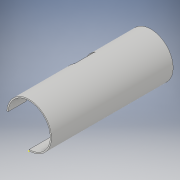
# Autodesk Inventor part: upperClaw
Saved by Autodesk Inventor 2017 (Build 210142000, 142)
## iProperties
Created: 2017-04-06
Part Number: upperClaw
Material: Generic
Document SubType Name: Modeling
Designer: s4461999
Density: 1 g/cm^3
Appearance: Default
Author: s4461999
Autodesk Inventor part; units mm, degrees
ref_plane "YZ Plane" through (0, 0, 0) normal (1, 0, 0) x (0, 1, 0)
ref_plane "XZ Plane" through (0, 0, 0) normal (0, 1, 0) x (-1, 0, 0)
ref_plane "XY Plane" through (0, 0, 0) normal (0, 0, 1) x (1, 0, 0)
sketch "Sketch1" plane through (0, 0, 0) normal (0, 0, 1) x (1, 0, 0)
  point P0 (0, 0)
sketch "Sketch2" plane through (0, 0, 0) normal (0, 0, 1) x (1, 0, 0)
  line L0 (0, 0) -> (0, 3)
  arc A0 (0, 3) -> (-49.4537, 71.0727) centre (0, 55) ccw
  arc A1 (0, 0) -> (-52.3068, 72) centre (0, 55) ccw
  line L1 (-52.3068, 72) -> (-49.4537, 71.0727)
  dimension "d16" = 55
  dimension "d17" = 52
  dimension "d18" = 0
  dimension "d20" = 72
  constraints: 4 end point, 4 point on circle, 2 centre point, 1 coincident, 1 line through centre, 1 vertical
  measures "d16" radius of A1
  measures "d17" radius of A0
  measures "d18" distance from line of L0 A0.centre
  measures "d20" vertical distance of L0.start L1.start
extrude "Extrusion1" add sketch "Sketch2" along normal blind 300
sketch "Sketch3" plane through (0, 0, 0) normal (0, 0, -1) x (-1, 0, 0)
  arc A0 (52.3068, 72) -> (0, 0) centre (0, 55) ccw projected
  line L0 (0, 55) -> (57.5671, 81.8494)
  line L1 (49.4537, 71.0727) -> (52.3068, 72) projected
  dimension "d25" = 7
  constraints: 2 end point
  measures "d25" angle of L0 L1
sketch "Sketch4" plane through (0, 0, 0) normal (0, 0, -1) x (-1, 0, 0)
  point P0 (0, 0)
sketch "Sketch5" plane through (0, 0, 300) normal (0, 0, 1) x (1, 0, 0)
  point P0 (0, 0)
ref_plane "Work Plane1" through (-49.8451, 78.2479, 0) normal (-0.9062749, 0.4226887, 0) x (-0.4226887, -0.9062749, 0)
sketch "Sketch6" plane through (-49.8451, 78.2479, 0) normal (-0.9062749, 0.4226887, 0) x (-0.4226887, -0.9062749, 0)
  line L0 (-91.8755, 150) -> (67.0312, 150)
  line L1 (-55, 0) -> (49.8451, 0) projected
  line L2 (6.7028, 0) -> (6.7028, 300) projected
  point P0 (-0.0122, 59)
  point P1 (-0.0122, 93)
  point P2 (-0.0122, 241)
  point P3 (-0.0122, 207)
  dimension "d26" = 150
  dimension "d27" = 57
  dimension "d28" = 34
  dimension "d29" = 6.715
  dimension "d30" = 6.715
  constraints: 2 end point, 2 symmetric about line, 1 horizontal
  measures "d26" distance between parallel lines of L0 L1
  measures "d27" distance from line of point (-0.012, 93) L0
  measures "d28" distance of point (-0.012, 59) point (-0.012, 93)
  measures "d29" distance from line of L2 point (-0.012, 59)
  measures "d30" distance from line of L2 point (-0.012, 93)
hole "Hole1" at (-49.84, 78.2589, 59) at (-49.84, 78.2589, 93) at (-49.84, 78.2589, 207) at (-49.84, 78.2589, 241) direction (0.9062749, -0.4226887, 0) diameter 4.4 depth 8 tip angle 118
sketch "Sketch7" plane through (-49.8451, 78.2479, 0) normal (-0.9062749, 0.4226887, 0) x (-0.4226887, -0.9062749, 0)
  line L0 (-33, 110.2) -> (13, 110.2)
  line L1 (13, 110.2) -> (13, 160.2)
  line L2 (13, 160.2) -> (-33, 160.2)
  line L3 (-33, 160.2) -> (-33, 110.2)
  point P0 (49.8451, 0)
  point P1 (0, 95.2)
  dimension "d38" = 50
  dimension "d39" = 15
  dimension "d41" = 33
  constraints: 8 end point, 2 parallel, 1 horizontal, 1 perpendicular
  measures "d38" distance of L0.end L1.end
  measures "d39" distance from line of L0 point (0, 95.2)
  measures "d41" distance from line of L3 point (0, 95.2)
extrude "Extrusion2" cut sketch "Sketch7" against normal blind 10
sketch "Sketch8" plane through (0, 55, 110.2) normal (0, 0, 1) x (0.7765651, -0.630037, 0)
  point P0 (34.652, -42.7111)
sketch "Sketch9" plane through (0, 55, 110.2) normal (0, 0, 1) x (0.7765651, -0.630037, 0)
  point P0 (34.652, -42.7111)
ref_plane "Work Plane2" through (-27.4158, 102.6799, 0) normal (-0.4984688, 0.8669077, 0) x (-0.8669077, -0.4984688, 0)
sketch "Sketch10" plane through (-27.4158, 102.6799, 0) normal (-0.4984688, 0.8669077, 0) x (-0.8669077, -0.4984688, 0)
  line L0 (0, 110.2) -> (36.8712, 110.2) projected
  line L1 (4.5533, 160.2) -> (34.86, 160.2) projected
  line L2 (0, 110.2) -> (4.5533, 110.2)
  line L3 (4.5533, 110.2) -> (4.5533, 160.2)
  line L4 (4.5533, 160.2) -> (0, 160.2)
  line L5 (0, 160.2) -> (0, 110.2)
  point P0 (27.4158, 0)
  constraints: 8 end point, 2 parallel, 1 horizontal, 1 perpendicular
extrude "Extrusion3" cut sketch "Sketch10" against normal blind 10
sketch "Sketch12" plane through (0, 0, 0) normal (0, 0, -1) x (-1, 0, 0)
  line L0 (49.4537, 71.0727) -> (52.3068, 72) projected
  arc A0 (51.9285, 57.7255) -> (49.4537, 71.0727) centre (0, 55) ccw
  arc A1 (54.9244, 57.8827) -> (52.3068, 72) centre (0, 55) ccw
  line L1 (52.3068, 72) -> (49.4537, 71.0727)
  line L2 (54.9244, 57.8827) -> (51.9285, 57.7255)
  point P0 (0, 0)
  dimension "d47" = 52
  dimension "d48" = 55
  dimension "d49" = 15
  constraints: 4 end point, 4 point on circle, 2 centre point, 1 concentric, 1 line through centre
  measures "d47" radius of A0
  measures "d48" radius of A1
extrude "Extrusion4" add sketch "Sketch12" against normal blind 45
ref_plane "Work Plane3" through (0, 0, 150) normal (0, 0, -1) x (-1, 0, 0)
mirror "Mirror1" about plane through (0, 0, 150) normal (0, 0, -1) of "Extrusion4"
body "Solid1"
